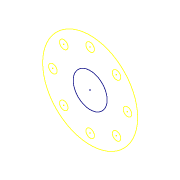
# Autodesk Inventor part: bar2
Saved by Autodesk Inventor 2020 (Build 240168000, 168)
## iProperties
Created: 2020-11-05
Part Number: bar2
Material: 일반
Document SubType Name: Sheet Metal
Designer: 이호석
Mass: 23.7671 g
Surface Area: 142.542 cm^2
Volume: 23.7671 cm^3
Density: 1 g/cm^3
Sheet Metal Rule: 기본값
Appearance: 기본값
Author: 이호석
Autodesk Inventor part; units mm, degrees
ref_plane "YZ Plane" through (0, 0, 0) normal (1, 0, 0) x (0, 1, 0)
ref_plane "XZ Plane" through (0, 0, 0) normal (0, 1, 0) x (-1, 0, 0)
ref_plane "XY Plane" through (0, 0, 0) normal (0, 0, 1) x (1, 0, 0)
sketch "스케치1" plane through (0, 0, 0) normal (0, 0, 1) x (1, 0, 0)
  circle A0 centre (7.7782, 7.7782) radius 1.25
  circle A1 centre (-7.7782, 7.7782) radius 1.25
  circle A2 centre (7.7782, -7.7782) radius 1.25
  circle A3 centre (-11, 0) radius 1.25
  circle A4 centre (11, 0) radius 1.25
  circle A5 centre (0, 11) radius 1.25
  circle A6 centre (0, -11) radius 1.25
  circle A7 centre (-7.7782, -7.7782) radius 1.25
  circle A8 centre (0, 0) radius 14
  circle A9 centre (0, 0) radius 5
  circle A10 centre (0, 0) radius 5
  line L0 (5, 0) -> (5, -10)
  line L1 (5, -10) -> (-5, -10)
  line L2 (-5, -10) -> (-5, 0)
  line L3 (15, -10) -> (-15, -10)
  line L4 (-15, -10) -> (-15, 195)
  line L5 (-15, 195) -> (15, 195)
  line L6 (15, 195) -> (15, -10)
  line L7 (0, 195) -> (0, 165)
  line L8 (0, 165) -> (4.2095, 175.1627)
  line L9 (0, 165) -> (11, 165) construction
  circle A11 centre (4.2095, 175.1627) radius 1.25
  circle A12 centre (-4.2095, 175.1627) radius 1.25
  circle A13 centre (-10.1627, 169.2095) radius 1.25
  circle A14 centre (-10.1627, 160.7905) radius 1.25
  circle A15 centre (-4.2095, 154.8373) radius 1.25
  circle A16 centre (4.2095, 154.8373) radius 1.25
  circle A17 centre (10.1627, 160.7905) radius 1.25
  circle A18 centre (10.1627, 169.2095) radius 1.25
  dimension "d0" = 10
  dimension "d2" = 30
  dimension "d3" = 205
  dimension "d4" = 30
  dimension "d6" = 11
  dimension "d7" = 67.5
  dimension "d8" = 2.5
  dimension "d11" = 360
  measures "d0" distance of L0.start L0.end
  measures "d2" distance of L4.end L5.end
  measures "d3" distance of L3.end L4.end
  measures "d4" distance of L7.start L7.end
  measures "d6" distance of L8.start L8.end
  measures "d7" angle of L9 L8
  measures "d8" diameter of A11
extrude "판1" add sketch "스케치1" along normal blind 4 contours L0 A9 L2 L3 A8 | A8 L3 L4 L5 L6 | A15 | A16
fillet "모서리 라운드1" radius 2 6 edges at (15, -10, 2) (5, -10, 2) (-5, -10, 2) (-15, -10, 2) (15, 195, 2) (-15, 195, 2)
equation "\"TransitionRadius\" = BendRadius"
equation "\"BendRadius\" = 4"
